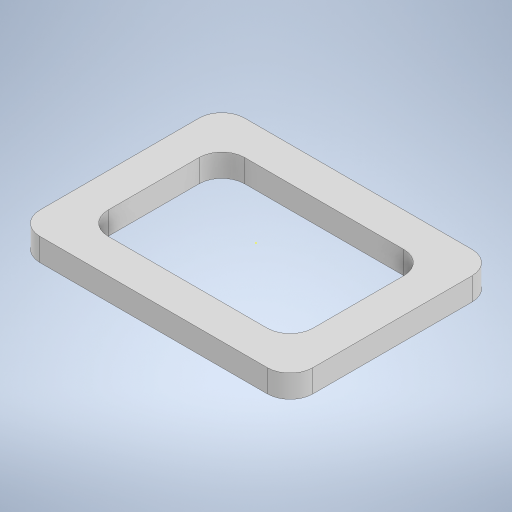
# Autodesk Inventor part: Spacer
Saved by Autodesk Inventor 2024 (Build 280153000, 153)
## iProperties
Created: 2024-05-15
Part Number: Spacer
Material: Generic
Document SubType Name: Modeling
Designer: andre
Density: 1 g/cm^3
Appearance: Default
Author: andre
## iProperties of the stored document Spacer_3DPrint.ipt
Created: 2024-05-15
Part Number: Spacer_3DPrint
Material: Generic
Document SubType Name: Modeling
Designer: andre
Density: 1 g/cm^3
Appearance: Default
Author: andre
Autodesk Inventor part; units mm, degrees
ref_plane "YZ Plane" through (0, 0, 0) normal (1, 0, 0) x (0, 1, 0)
ref_plane "XZ Plane" through (0, 0, 0) normal (0, 1, 0) x (-1, 0, 0)
ref_plane "XY Plane" through (0, 0, 0) normal (0, 0, 1) x (1, 0, 0)
sketch "Sketch1" plane through (0, 0, 0) normal (0, 1, 0) x (-1, 0, 0)
  line L0 (6, 4.5) -> (-6, 4.5)
  line L1 (-6, 4.5) -> (-6, -4.5)
  line L2 (-6, -4.5) -> (6, -4.5)
  line L3 (6, -4.5) -> (6, 4.5)
  line L4 (6, 4.5) -> (-6, -4.5) construction
  line L5 (-6, 4.5) -> (6, -4.5) construction
  point P0 (0, 0)
  dimension "d4" = 12
  dimension "d5" = 9
  constraints: 12 end point, 2 midpoint, 2 parallel, 1 horizontal, 1 perpendicular
  measures "d4" distance of L2.end L1.end
  measures "d5" distance of L1.end L0.end
extrude "Extrusion1" add sketch "Sketch1" along normal blind 1
sketch "Sketch2" plane through (0, 1, 0) normal (0, 1, 0) x (1, 0, 0)
  point P0 (0, 0)
fillet "Fillet1" radius 1 4 edges at (6, 0.5, 4.5) (6, 0.5, -4.5) (-6, 0.5, -4.5) (-6, 0.5, 4.5)
sketch "Sketch3" plane through (0, 1, 0) normal (0, 1, 0) x (1, 0, 0)
  arc A0 (-6, -3.5) -> (-5, -4.5) centre (-5, -3.5) ccw projected
  line L0 (-5, -4.5) -> (5, -4.5) projected
  arc A1 (5, -4.5) -> (6, -3.5) centre (5, -3.5) ccw projected
  line L1 (6, -3.5) -> (6, 3.5) projected
  arc A2 (6, 3.5) -> (5, 4.5) centre (5, 3.5) ccw projected
  line L2 (5, 4.5) -> (-5, 4.5) projected
  arc A3 (-5, 4.5) -> (-6, 3.5) centre (-5, 3.5) ccw projected
  line L3 (-6, 3.5) -> (-6, -3.5) projected
  line L4 (-4.5, -3) -> (4.5, -3)
  line L5 (4.5, -3) -> (4.5, 3)
  line L6 (4.5, 3) -> (-4.5, 3)
  line L7 (-4.5, 3) -> (-4.5, -3)
  point P0 (0, 0)
  dimension "d7" = 1.5
  constraints: 8 end point, 3 other
  measures "d7" distance between parallel lines of L3 L7
extrude "Extrusion2" cut sketch "Sketch3" against normal up to next contours L7 L6 L5 L4
fillet "Fillet2" radius 1 4 edges at (-4.5, 0.5, 3) (-4.5, 0.5, -3) (4.5, 0.5, 3) (4.5, 0.5, -3)
body "Solid1"
